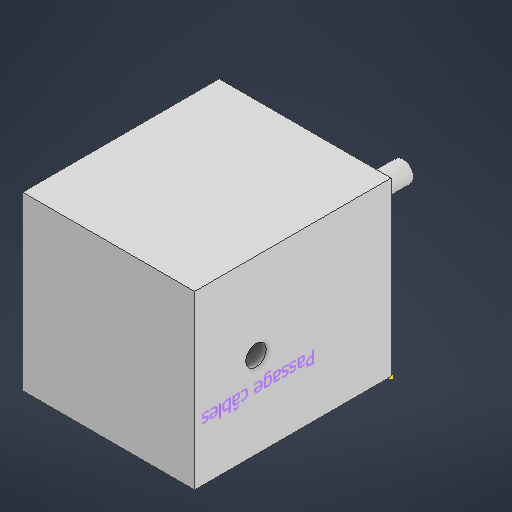
# Autodesk Inventor part: moteur 17HS19-2004S1
Saved by Autodesk Inventor 2026.2 (Build 302298010, 298A)
## iProperties
Created: 2026-03-17
Part Number: moteur 17HS19-2004S1
Material: Générique
Document SubType Name: Modeling
Designer: cleml
Density: 1 g/cm^3
Appearance: Par défaut
Author: cleml
Autodesk Inventor part; units mm, degrees
ref_plane "YZ Plane" through (0, 0, 0) normal (1, 0, 0) x (0, 1, 0)
ref_plane "XZ Plane" through (0, 0, 0) normal (0, 1, 0) x (-1, 0, 0)
ref_plane "XY Plane" through (0, 0, 0) normal (0, 0, 1) x (1, 0, 0)
sketch "Esquisse1" plane through (0, 0, 0) normal (0, 0, 1) x (1, 0, 0)
  line L0 (0, 0) -> (42, 0)
  line L1 (42, 0) -> (42, 42)
  line L2 (42, 42) -> (0, 42)
  line L3 (0, 42) -> (0, 0)
  dimension "d0" = 42
  dimension "d1" = 42
  constraints: 8 end point, 2 parallel, 1 horizontal, 1 perpendicular
  measures "d0" distance of L1.end L2.end
  measures "d1" distance of L0.end L1.end
extrude "Extrusion1" add sketch "Esquisse1" along normal blind 48
sketch "Esquisse2" plane through (0, 0, 0) normal (0, 0, -1) x (-1, 0, 0)
  line L0 (0, 42) -> (0, 0) projected
  line L1 (0, 0) -> (-42, 0) projected
  circle A0 centre (-21, 21) radius 12.5
  dimension "d4" = 21
  dimension "d5" = 21
  dimension "d6" = 25
  constraints: 1 centre point, 1 coincident
  measures "d4" distance from line of L0 point (-21, 21)
  measures "d5" distance from line of L1 point (-21, 21)
  measures "d6" diameter of A0
extrude "Extrusion2" cut sketch "Esquisse2" against normal blind 2
sketch "Esquisse5" plane through (21, 21, 2) normal (0, 0, -1) x (-1, 0, 0)
  circle A0 centre (0, 0) radius 12.5 projected
  circle A1 centre (0, 0) radius 3.5
  point P0 (21, -21)
  dimension "d18" = 7
  constraints: 1 centre point, 1 coincident
  measures "d18" diameter of A1
extrude "Extrusion5" cut sketch "Esquisse5" against normal blind 15 contours A1
sketch "Esquisse6" plane through (21, 21, 17) normal (0, 0, -1) x (-1, 0, 0)
  circle A0 centre (0, 0) radius 3.5 projected
  circle A1 centre (0, 0) radius 2.5
  point P0 (21, -21)
  dimension "d21" = 5
  constraints: 1 centre point, 1 coincident
  measures "d21" diameter of A1
extrude "Extrusion6" add sketch "Esquisse6" along normal blind 41 contours A1
sketch "Esquisse7" plane through (42, 0, 0) normal (1, 0, 0) x (0, 0, -1)
  line L0 (0, 0) -> (-48, 0) projected
  line L1 (-48, 0) -> (-48, 42) projected
  circle A0 centre (-33, 21) radius 2.5
  line L2 (-15.5634, 24.7779) -> (-36.4192, 24.7779) construction
  line L3 (-36.4192, 24.7779) -> (-36.4192, 35.8396) construction
  line L4 (-36.4192, 35.8396) -> (-15.5634, 35.8396) construction
  line L5 (-15.5634, 35.8396) -> (-15.5634, 24.7779) construction
  dimension "d24" = 21
  dimension "d25" = 15
  dimension "d26" = 5
  constraints: 1 centre point, 1 coincident, 2 other
  measures "d24" distance from line of L0 point (-33, 21)
  measures "d25" distance from line of L1 point (-33, 21)
  measures "d26" diameter of A0
extrude "Extrusion7" cut sketch "Esquisse7" against normal blind 20
sketch "Esquisse8" plane through (42, 0, 0) normal (1, 0, 0) x (0, 0, -1)
  line L0 (-18.5513, 11.8106) -> (-48.2794, 11.8106) construction
  line L1 (-48.2794, 11.8106) -> (-48.2794, 27.9421) construction
  line L2 (-48.2794, 27.9421) -> (-18.5513, 27.9421) construction
  line L3 (-18.5513, 27.9421) -> (-18.5513, 11.8106) construction
  point P0 (0, 0)
  constraints: 2 other
